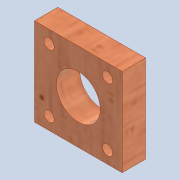
# Autodesk Inventor part: 0005-10-006 Capac rulment
Saved by Autodesk Inventor 2020 (Build 240168000, 168)
## iProperties
Created: 2020-12-18
Part Number: 0005-10-006 Capac rulment
Material: Generic
Document SubType Name: Modeling
Designer: Iulian Bors
Density: 1 g/cm^3
Appearance: White Oak - Natural Medium Gloss
Author: Iulian Bors
Subject: 006
Autodesk Inventor part; units mm, degrees
ref_plane "YZ Plane" through (0, 0, 0) normal (1, 0, 0) x (0, 1, 0)
ref_plane "XZ Plane" through (0, 0, 0) normal (0, 1, 0) x (-1, 0, 0)
ref_plane "XY Plane" through (0, 0, 0) normal (0, 0, 1) x (1, 0, 0)
sketch "Sketch1" plane through (0, 0, 0) normal (0, 0, 1) x (1, 0, 0)
  line L0 (-15, 15) -> (15, 15)
  line L1 (15, 15) -> (15, -15)
  line L2 (15, -15) -> (-15, -15)
  line L3 (-15, -15) -> (-15, 15)
  point P0 (0, 0)
  point P1 (0, 15)
  point P2 (-15, 0)
  dimension "d0" = 30
  dimension "d1" = 30
  constraints: 8 end point, 2 midpoint, 2 parallel, 1 horizontal, 1 horizontal alignment, 1 perpendicular, 1 vertical alignment
  measures "d0" distance of L0.start L0.end
  measures "d1" distance of L2.end L0.start
extrude "Extrusion1" add sketch "Sketch1" along normal blind 8
sketch "Sketch2" plane through (0, 0, 8) normal (0, 0, 1) x (1, 0, 0)
  circle A0 centre (0, 0) radius 7.5
  line L0 (15, 15) -> (-15, 15) projected
  line L1 (-15, 15) -> (-15, -15) projected
  point P0 (0, 15)
  point P1 (-15, 0)
  dimension "d17" = 15
  constraints: 2 midpoint, 1 centre point, 1 horizontal alignment, 1 vertical alignment
  measures "d17" diameter of A0
extrude "Extrusion2" cut sketch "Sketch2" against normal through all
sketch "Sketch3" plane through (0, 0, 8) normal (0, 0, 1) x (1, 0, 0)
  circle A0 centre (10, -10.75) radius 1.75
  circle A1 centre (10, 10.75) radius 1.75
  line L0 (15, 15) -> (-15, 15) projected
  line L1 (15, -15) -> (15, 15) projected
  circle A2 centre (-10, -10.75) radius 1.75
  circle A3 centre (-10, 10.75) radius 1.75
  line L2 (-15, 15) -> (-15, -15) projected
  line L3 (-15, -15) -> (15, -15) projected
  line L4 (10, 10.75) -> (-10, 10.75) construction
  line L5 (-10, 10.75) -> (-10, -10.75) construction
  line L6 (-10, -10.75) -> (10, -10.75) construction
  line L7 (10, -10.75) -> (10, 10.75) construction
  point P0 (0, 0)
  point P1 (10, 0)
  point P2 (0, 10.75)
  dimension "d9" = 3.5
  dimension "d19" = 10.75
  dimension "d20" = 10.75
  dimension "d21" = 20
  dimension "d22" = 21.5
  constraints: 8 end point, 4 centre point, 3 coincident, 3 equal radius, 3 horizontal alignment, 3 vertical alignment, 2 midpoint, 2 parallel, 1 horizontal, 1 perpendicular
  measures "d9" diameter of A0
  measures "d19" vertical distance of A0.centre point (0, 0)
  measures "d20" vertical distance of point (0, 0) A1.centre
  measures "d21" distance of L4.start L4.end
  measures "d22" distance of L6.end L4.start
extrude "Extrusion3" cut sketch "Sketch3" against normal through all contours A0 | A1 | A2 | A3
body "Solid1"
